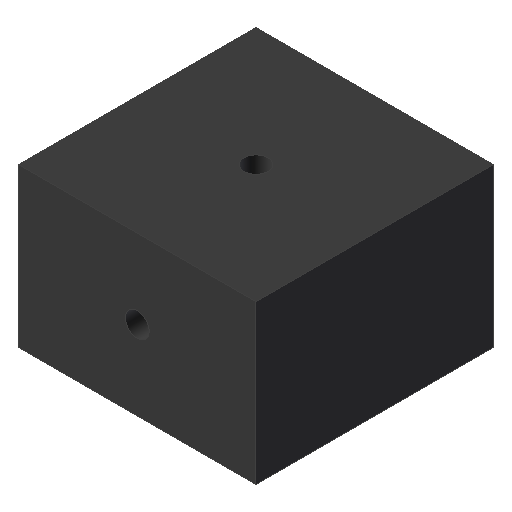
# Autodesk Inventor part: fengmingroboticarm2
Saved by Autodesk Inventor 2025 (Build 290162000, 162)
## iProperties
Created: 2025-02-16
Part Number: fengmingroboticarm2
Material: Generic
Document SubType Name: Modeling
Designer: wj
Density: 1 g/cm^3
Appearance: Default
Author: wj
Autodesk Inventor part; units mm, degrees
ref_plane "YZ Plane" through (0, 0, 0) normal (1, 0, 0) x (0, 1, 0)
ref_plane "XZ Plane" through (0, 0, 0) normal (0, 1, 0) x (-1, 0, 0)
ref_plane "XY Plane" through (0, 0, 0) normal (0, 0, 1) x (1, 0, 0)
sketch "Sketch1" plane through (0, 0, 0) normal (0, 1, 0) x (-1, 0, 0)
  line L0 (1.6133, 19.7766) -> (-28.3867, 19.7766)
  line L1 (-28.3867, 19.7766) -> (-28.3867, -10.2234)
  line L2 (-28.3867, -10.2234) -> (1.6133, -10.2234)
  line L3 (1.6133, -10.2234) -> (1.6133, 19.7766)
  point P0 (0, 0)
  dimension "d0" = 30
  dimension "d1" = 30
  constraints: 8 end point, 2 parallel, 1 horizontal, 1 perpendicular
  measures "d0" distance of L2.end L1.end
  measures "d1" distance of L0.end L1.end
extrude "Extrusion1" add sketch "Sketch1" along normal blind 20
sketch "Sketch2" plane through (-1.6133, 0, 19.7766) normal (0, 0, 1) x (1, 0, 0)
  circle A0 centre (15, 10) radius 1.5
  line L0 (0, 0) -> (30, 0) projected
  line L1 (0, 0) -> (0, 20) projected
  point P0 (1.6133, 0)
  point P1 (0, 10)
  dimension "d4" = 3
  dimension "d5" = 10
  dimension "d6" = 15
  constraints: 1 centre point, 1 midpoint
  measures "d4" diameter of A0
  measures "d5" distance from line of L0 A0.centre
  measures "d6" distance of point (0, 10) A0.centre
extrude "Extrusion2" cut sketch "Sketch2" against normal blind 500
sketch "Sketch3" plane through (0, 20, 0) normal (0, 1, 0) x (1, 0, 0)
  circle A0 centre (13.3867, -4.7766) radius 1.5
  line L0 (28.3867, -19.7766) -> (28.3867, 10.2234) projected
  line L1 (28.3867, 10.2234) -> (-1.6133, 10.2234) projected
  point P0 (0, 0)
  dimension "d9" = 3
  dimension "d10" = 15
  dimension "d11" = 15
  constraints: 1 centre point
  measures "d9" diameter of A0
  measures "d10" distance from line of L0 A0.centre
  measures "d11" distance from line of L1 A0.centre
extrude "Extrusion3" cut sketch "Sketch3" against normal blind 500
body "Solid1"
